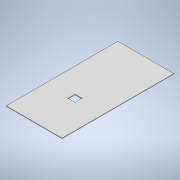
# Autodesk Inventor part: left
Saved by Autodesk Inventor 2021 (Build 250183000, 183)
## iProperties
Created: 2021-03-25
Part Number: left
Material: Generic
Document SubType Name: Modeling
Designer: noori
Density: 1 g/cm^3
Appearance: Default
Author: noori
Autodesk Inventor part; units mm, degrees
ref_plane "YZ Plane" through (0, 0, 0) normal (1, 0, 0) x (0, 1, 0)
ref_plane "XZ Plane" through (0, 0, 0) normal (0, 1, 0) x (-1, 0, 0)
ref_plane "XY Plane" through (0, 0, 0) normal (0, 0, 1) x (1, 0, 0)
sketch "Sketch1" plane through (0, 0, 0) normal (0, 1, 0) x (-1, 0, 0)
  line L0 (200, 400) -> (-200, 400)
  line L1 (-200, 400) -> (-200, -400)
  line L2 (-200, -400) -> (200, -400)
  line L3 (200, -400) -> (200, 400)
  line L4 (25, 132) -> (-25, 132)
  line L5 (-25, 132) -> (-25, 82)
  line L6 (-25, 82) -> (25, 82)
  line L7 (25, 82) -> (25, 132)
  point P0 (0, 0)
  dimension "d0" = 800
  dimension "d1" = 400
  dimension "d2" = 50
  dimension "d3" = 50
  dimension "d4" = 175
  dimension "d5" = 268
  dimension "d7" = 200
  dimension "d8" = 400
  constraints: 16 end point, 4 parallel, 2 horizontal, 2 perpendicular
  measures "d0" distance of L2.end L0.start
  measures "d1" distance of L0.start L0.end
  measures "d2" distance of L6.end L4.start
  measures "d3" distance of L5.end L6.end
  measures "d4" distance between parallel lines of L3 L7
  measures "d5" distance between parallel lines of L0 L4
  measures "d7" distance from line of L3 point (0, 0)
  measures "d8" distance from line of L0 point (0, 0)
extrude "Extrusion1" add sketch "Sketch1" along normal mid plane 4
body "Solid1"
